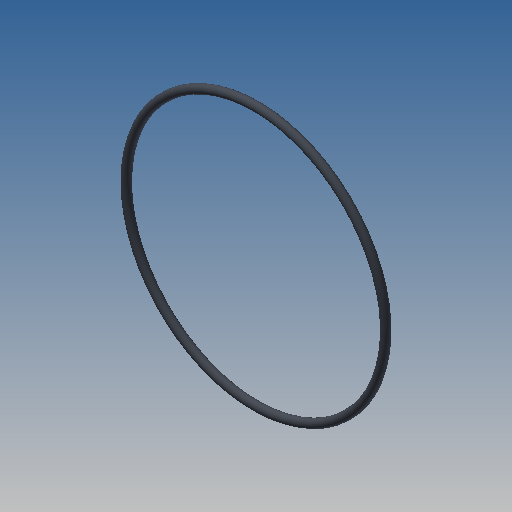
# Autodesk Inventor part: 9452K194
Saved by Autodesk Inventor 2018.2 (Build 222227000, 227)
## iProperties
Created: 2014-04-04
Material: VERO BLACK
Vendor: MCMASTER
Document SubType Name: Modeling
Designer: NEGRASHOVI
Mass: 247.244 g
Surface Area: 1522.49 cm^2
Volume: 211.319 cm^3
Density: 1.17 g/cm^3
Description: O-RING DASH 244
Project: COMMON
Appearance: Black Anodize
Part Number: 9452K194
RuleStatus: InUse
AfterDocSave0: file://Part Number Cleaner
LAB/DEPT: COMMON
REQUESTING SCIENTIST: COMMON
SURFACE ROUGHNESS: N/A
DESIGN DEPARTMENT: HHMI: JRC - ID&F
SPECIAL FINISH: NONE
ALTERED ITEM PART NUMBER: N/A
ALTERED ITEM VENDOR: N/A
ALTERED ITEM DESCRIPTION: N/A
Author: NEGRASHOVI
Revision Number: -
Autodesk Inventor part; units mm, degrees
ref_plane "YZ Plane" through (0, 0, 0) normal (1, 0, 0) x (0, 1, 0)
ref_plane "XZ Plane" through (0, 0, 0) normal (0, 1, 0) x (-1, 0, 0)
ref_plane "XY Plane" through (0, 0, 0) normal (0, 0, 1) x (1, 0, 0)
sketch "Sketch12" plane through (0, 0, 0) normal (1, 0, 0) x (0, 1, 0)
  circle A0 centre (-55.5371, 0) radius 1.7653
  line L0 (0, -2.4714) -> (0, 2.4714) construction
  point P0 (0, 0)
  dimension "d70" = 3.5306
  dimension "d71" = 114.6048
  constraints: 1 centre point, 1 horizontal alignment
  measures "d70" diameter of A0
revolve "Revolution2" add sketch "Sketch12" angle 360 about axis through (0, 0, -10) along (0, 0, 1)
body "Solid1"
